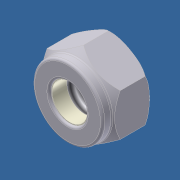
# Autodesk Inventor part: HW-00033
Saved by Autodesk Inventor 2012 (Build 160160000, 160)
## iProperties
Created: 2008-10-27
Part Number: HW-00033
Material: Steel
Description: Nut, Nylock 5/16-18 Zinc Plate
Document SubType Name: Modeling
Designer: firstuser
Mass: 6.30581 g
Surface Area: 6.79186 cm^2
Volume: 0.803287 cm^3
Density: 7.85 g/cm^3
Title: Nut, Nylock 5/16-18 Zinc Plate
Author: firstuser
Autodesk Inventor part; units mm, degrees
ref_plane "YZ Plane" through (0, 0, 0) normal (1, 0, 0) x (0, 1, 0)
ref_plane "XZ Plane" through (0, 0, 0) normal (0, 1, 0) x (-1, 0, 0)
ref_plane "XY Plane" through (0, 0, 0) normal (0, 0, 1) x (1, 0, 0)
sketch "Sketch1" plane through (0, 0, 0) normal (0, 0, 1) x (1, 0, 0)
  line L0 (0, 7.3323) -> (6.35, 3.6662)
  line L1 (6.35, 3.6662) -> (6.35, -3.6662)
  line L2 (6.35, -3.6662) -> (0, -7.3323)
  line L3 (0, -7.3323) -> (-6.35, -3.6662)
  line L4 (-6.35, -3.6662) -> (-6.35, 3.6662)
  line L5 (-6.35, 3.6662) -> (0, 7.3323)
  line L6 (0, 10.2653) -> (0, -10.2653) projected
  line L7 (-8.89, 0) -> (8.89, 0) projected
  point P0 (0, 0)
  dimension "d0" = 12.7
  constraints: 12 end point, 2 midpoint, 1 vertical, 13 other
  measures "d0" distance between parallel lines of L1 L4
extrude "Extrusion1" add sketch "Sketch1" along normal blind 7.8486
sketch "Sketch2" plane through (0, 0, 0) normal (1, 0, 0) x (0, 1, 0)
  line L0 (7.3323, 0) -> (7.3323, 7.8486) projected
  line L1 (3.6662, 7.8486) -> (-3.6662, 7.8486) projected
  line L2 (7.3323, 7.8486) -> (3.6662, 7.8486) projected
  line L3 (3.6662, 7.8486) -> (7.3323, 7.8486) projected
  line L4 (-3.6662, 7.8486) -> (3.6662, 7.8486) projected
  line L5 (-7.3323, 7.8486) -> (-3.6662, 7.8486) projected
  line L6 (-3.6662, 7.8486) -> (-7.3323, 7.8486) projected
  line L7 (7.3323, 5.0546) -> (6.096, 6.2909)
  line L8 (6.096, 6.2909) -> (6.096, 7.8486)
  line L9 (7.3323, 7.8486) -> (7.3323, 5.0546)
  line L10 (5.588, 7.4676) -> (3.048, 7.4676)
  line L11 (3.048, 7.4676) -> (3.048, 4.9276)
  line L12 (3.048, 4.9276) -> (5.588, 4.9276)
  line L13 (5.588, 4.9276) -> (5.588, 7.4676)
  line L14 (0, 13.9621) -> (0, -2.3404) projected
  arc A0 (6.35, 0) -> (7.3323, 0.762) centre (5.3317, 2.327) ccw
  line L15 (7.3323, 0) -> (3.6662, 0) projected
  line L16 (6.35, 0) -> (7.3323, 0)
  line L17 (7.3323, 0.762) -> (7.3323, 0)
  dimension "d3" = 2.794
  dimension "d4" = 45
  dimension "d5" = 6.096
  dimension "d6" = 3.048
  dimension "d7" = 0.381
  dimension "d8" = 2.54
  dimension "d9" = 2.54
  dimension "d11" = 6.35
  dimension "d12" = 0.762
  dimension "d13" = 2.54
  constraints: 18 end point, 4 point on line, 3 perpendicular, 2 collinear, 2 parallel, 2 point on circle, 1 centre point, 1 horizontal
  measures "d3" distance of L0.end L7.start
  measures "d4" angle of L9 L7
  measures "d5" distance between parallel lines of L14 L8
  measures "d6" distance between parallel lines of L11 L14
  measures "d7" distance between parallel lines of L10 L2
  measures "d8" distance between parallel lines of L12 L10
  measures "d9" distance of L11.end L12.end
  measures "d11" distance from line of L14 L16.start
  measures "d12" distance of L17.start L0.start
  measures "d13" radius of A0
revolve "Revolution1" cut sketch "Sketch2" angle 360 about axis through (0, 0, 0) along (0, 0, -1) contours L7 L8 L2 L0
revolve "Revolution2" cut sketch "Sketch2" angle 360 about axis through (0, 0, 0) along (0, 0, -1) contours L15 A0 L0
hole "Hole1" at (0, 0, 7.8486) direction (0, 0, -1) diameter 6.4008 end through all thread size "5/16-18 UNC" class "2B" standard "ANSI Unified Screw Threads"
fillet "Fillet1" radius 0.381 3 edges at (0, -6.096, 6.2909) (0, -6.096, 7.8486) (0, 3.2004, 7.8486)
revolve "Revolution3" add sketch "Sketch2" angle 360 about axis through (0, 0, 0) along (0, 0, -1) contours L13 L12 L11 L10
body "Solid1"
